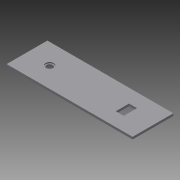
# Autodesk Inventor part: placa verticala priza
Saved by Autodesk Inventor 2015 SP1 (Build 190203100, 203)
## iProperties
Created: 2015-08-10
Part Number: placa verticala priza
Material: Generic
Document SubType Name: Modeling
Designer: ubik
Density: 1 g/cm^3
Appearance: Default
Author: ubik
Autodesk Inventor part; units mm, degrees
ref_plane "YZ Plane" through (0, 0, 0) normal (1, 0, 0) x (0, 1, 0)
ref_plane "XZ Plane" through (0, 0, 0) normal (0, 1, 0) x (-1, 0, 0)
ref_plane "XY Plane" through (0, 0, 0) normal (0, 0, 1) x (1, 0, 0)
sketch "Sketch1" plane through (0, 0, 0) normal (0, 0, 1) x (1, 0, 0)
  line L0 (-222.5, 72) -> (222.5, 72)
  line L1 (222.5, 72) -> (222.5, -72)
  line L2 (222.5, -72) -> (-222.5, -72)
  line L3 (-222.5, -72) -> (-222.5, 72)
  point P0 (0, 0)
  dimension "d0" = 445
  dimension "d1" = 144
  dimension "d2" = 72
  dimension "d3" = 222.5
  constraints: 8 end point, 2 parallel, 1 horizontal, 1 perpendicular
  measures "d0" distance of L1.end L2.end
  measures "d1" distance of L0.end L1.end
  measures "d2" distance from line of point (0, 0) L0
  measures "d3" distance from line of point (0, 0) L3
extrude "Extrusion1" add sketch "Sketch1" along normal blind 8
hole "Hole1" at (-142.5, 0, 8) direction (0, 0, -1) diameter 22 end through all
sketch "Sketch2" plane through (0, 0, 8) normal (0, 0, 1) x (1, 0, 0)
  circle A0 centre (-142.5, 0) radius 11 projected
  circle A1 centre (-142.5, 0) radius 14.5
  point P0 (0, 0)
  dimension "d15" = 29
  constraints: 1 centre point, 1 coincident
  measures "d15" diameter of A1
extrude "Extrusion2" cut sketch "Sketch2" against normal blind 4
sketch "Sketch3" plane through (0, 0, 8) normal (0, 0, 1) x (1, 0, 0)
  line L0 (114.5, 23.5) -> (142.5, 23.5)
  line L1 (142.5, 23.5) -> (142.5, -23.5)
  line L2 (142.5, -23.5) -> (114.5, -23.5)
  line L3 (114.5, -23.5) -> (114.5, 23.5)
  line L4 (222.5, -72) -> (222.5, 72) projected
  point P0 (0, 0)
  dimension "d18" = 28
  dimension "d19" = 47
  dimension "d20" = 80
  dimension "d21" = 23.5
  constraints: 8 end point, 2 parallel, 1 horizontal, 1 perpendicular
  measures "d18" distance of L1.end L2.end
  measures "d19" distance of L0.end L1.end
  measures "d20" distance between parallel lines of L4 L1
  measures "d21" distance from line of point (0, 0) L0
extrude "Extrusion3" cut sketch "Sketch3" against normal through all
equation "\"d2\" = 0.5 * d1"
equation "\"d3\" = 0.5 * d0"
equation "\"d21\" = 0.5 * d19"
body "Solid1"
